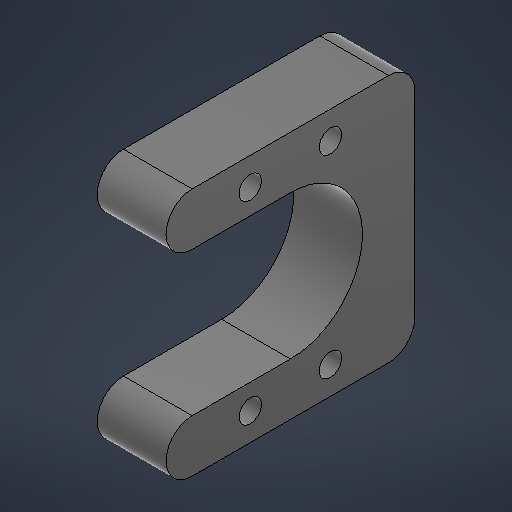
# Autodesk Inventor part: 3DPRINT,KICKER,MOTOR,MOUNT
Saved by Autodesk Inventor 2026.1 (Build 301233020, 233B)
## iProperties
Created: 2026-04-01
Part Number: 3DPRINT,KICKER,MOTOR,MOUNT
Material: Nylon 6/6
Document SubType Name: Modeling
Designer: Owen L
Mass: 36.9354 g
Surface Area: 101.53 cm^2
Volume: 32.6862 cm^3
Density: 1.13 g/cm^3
Appearance: Smooth - Black
Author: Owen L
Autodesk Inventor part; units mm, degrees
ref_plane "YZ Plane" through (0, 0, 0) normal (1, 0, 0) x (0, 1, 0)
ref_plane "XZ Plane" through (0, 0, 0) normal (0, 1, 0) x (-1, 0, 0)
ref_plane "XY Plane" through (0, 0, 0) normal (0, 0, 1) x (1, 0, 0)
sketch "Sketch2" plane through (0, 0, 0) normal (1, 0, 0) x (0, 1, 0)
  line L0 (30.1625, 30.1625) -> (30.1625, -30.1625)
  line L1 (30.1625, -30.1625) -> (-30.1625, -30.1625)
  line L2 (-30.1625, -30.1625) -> (-30.1625, 30.1625)
  line L3 (-30.1625, 30.1625) -> (30.1625, -30.1625) construction
  line L4 (30.1625, 30.1625) -> (-30.1625, -30.1625) construction
  arc A0 (-17.4625, 0) -> (17.4625, 0) centre (0, 0) ccw
  circle A1 centre (-23.4665, 9.7202) radius 2.7305
  circle A2 centre (-23.4665, -9.7202) radius 2.7305
  circle A3 centre (-9.7202, -23.4665) radius 2.7305
  circle A4 centre (9.7202, -23.4665) radius 2.7305
  circle A5 centre (23.4665, -9.7202) radius 2.7305
  circle A6 centre (23.4665, 9.7202) radius 2.7305
  circle A7 centre (9.7202, 23.4665) radius 2.7305
  circle A8 centre (-9.7202, 23.4665) radius 2.7305
  line L5 (-17.4625, 0) -> (-17.4625, 30.1625)
  line L6 (17.4625, 0) -> (17.4625, 30.1625)
  line L7 (-30.1625, 30.1625) -> (-17.4625, 30.1625)
  line L8 (17.4625, 30.1625) -> (30.1625, 30.1625)
  dimension "d14" = 25.4
  dimension "d19" = 34.925
  dimension "d20" = 60.325
  dimension "d21" = 5.461
  dimension "d24" = 360
  constraints: 18 end point, 9 centre point, 9 coincident, 7 perpendicular, 3 parallel, 2 horizontal, 2 midpoint, 2 point on circle, 2 tangent, 1 horizontal alignment, 25 other
  measures "d14" distance of point (0, 0) point (-23.467, 9.72)
  measures "d19" diameter of A0
  measures "d20" distance of L2.end L0.start
  measures "d21" diameter of A1
extrude "Extrusion1" add sketch "Sketch2" along normal blind 16.6675 contours L0 L1 L2 L7 L5 A0 L6 L8 | A3 | A4
fillet "Fillet1" radius 6.35 6 edges at (8.3337, 30.1625, -30.1625) (8.3337, 30.1625, 30.1625) (8.3337, 17.4625, 30.1625) (8.3337, -17.4625, 30.1625) (8.3337, -30.1625, 30.1625) (8.3337, -30.1625, -30.1625)
body "Solid1"
